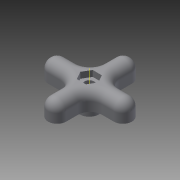
# Autodesk Inventor part: coil tightner
Saved by Autodesk Inventor 2013 (Build 170138000, 138)
## iProperties
Created: 2013-01-17
Part Number: coil tightner
Material: Generic
Document SubType Name: Modeling
Designer: Nico
Density: 1 g/cm^3
Author: Nico
Autodesk Inventor part; units mm, degrees
ref_plane "YZ Plane" through (0, 0, 0) normal (1, 0, 0) x (0, 1, 0)
ref_plane "XZ Plane" through (0, 0, 0) normal (0, 1, 0) x (-1, 0, 0)
ref_plane "XY Plane" through (0, 0, 0) normal (0, 0, 1) x (1, 0, 0)
sketch "Sketch1" plane through (0, 0, 0) normal (0, 0, 1) x (1, 0, 0)
  line L0 (17.5, 0) -> (27.5, 0)
  line L1 (35, 7.5) -> (35, 7.5)
  line L2 (27.5, 15) -> (17.5, 15)
  line L3 (0, 15) -> (0, 0)
  line L4 (-7.5, 7.5) -> (7.5, 7.5)
  line L5 (7.5, -10) -> (7.5, -20)
  line L6 (0, -27.5) -> (0, -27.5)
  line L7 (-7.5, -20) -> (-7.5, -10)
  line L8 (-17.5, 0) -> (-27.5, 0)
  line L9 (-35, 7.5) -> (-35, 7.5)
  line L10 (-27.5, 15) -> (-17.5, 15)
  line L11 (0, 15) -> (0, 0)
  line L12 (-7.5, 7.5) -> (7.5, 7.5)
  line L13 (7.5, 25) -> (7.5, 35)
  line L14 (0, 42.5) -> (0, 42.5)
  line L15 (-7.5, 35) -> (-7.5, 25)
  arc A0 (-17.5, 15) -> (-7.5, 25) centre (-17.5, 25) ccw
  arc A1 (7.5, 25) -> (17.5, 15) centre (17.5, 25) ccw
  arc A2 (17.5, 0) -> (7.5, -10) centre (17.5, -10) ccw
  arc A3 (-7.5, -10) -> (-17.5, 0) centre (-17.5, -10) ccw
  arc A4 (-27.5, 15) -> (-35, 7.5) centre (-27.5, 7.5) ccw
  arc A5 (-35, 7.5) -> (-27.5, 0) centre (-27.5, 7.5) ccw
  arc A6 (-7.5, -20) -> (0, -27.5) centre (0, -20) ccw
  arc A7 (0, -27.5) -> (7.5, -20) centre (0, -20) ccw
  arc A8 (27.5, 0) -> (35, 7.5) centre (27.5, 7.5) ccw
  arc A9 (35, 7.5) -> (27.5, 15) centre (27.5, 7.5) ccw
  arc A10 (7.5, 35) -> (0, 42.5) centre (0, 35) ccw
  arc A11 (0, 42.5) -> (-7.5, 35) centre (0, 35) ccw
  point P0 (35, 0)
  point P1 (7.5, -27.5)
  point P2 (-35, 0)
  point P3 (7.5, 42.5)
  dimension "d0" = 35
  dimension "d1" = 15
  dimension "d2" = 15
  dimension "d3" = 7.5
  dimension "d4" = 7.5
  dimension "d5" = 35
  dimension "d6" = 35
  dimension "d7" = 35
  dimension "d8" = 10
  dimension "d9" = 7.5
  constraints: 32 end point, 24 point on circle, 24 tangent, 16 point on line, 12 centre point, 10 equal radius, 8 parallel, 4 horizontal, 4 perpendicular
  measures "d0" distance of L3.end point (35, 0)
  measures "d1" distance of L3.start L3.end
  measures "d2" distance of L4.start L4.end
  measures "d3" distance between parallel lines of L5 L3
  measures "d4" distance between parallel lines of L0 L4
  measures "d5" distance of L4.end point (7.5, -27.5)
  measures "d6" distance of L3.end point (-35, 0)
  measures "d7" distance of L12.end point (7.5, 42.5)
  measures "d8" radius of A0
  measures "d9" radius of A4
extrude "Extrusion1" add sketch "Sketch1" along normal blind 15
sketch "Sketch2" plane through (0, 0, 15) normal (0, 0, 1) x (1, 0, 0)
  circle A0 centre (0, 6.9274) radius 3.95
  point P0 (0, 0)
  dimension "d12" = 7.9
  constraints: 1 centre point
  measures "d12" diameter of A0
extrude "Extrusion2" cut sketch "Sketch2" against normal blind 15
sketch "Sketch3" plane through (0, 0, 15) normal (0, 0, 1) x (1, 0, 0)
  circle A0 centre (0, 6.9274) radius 3.95 projected
  line L0 (-3.7206, 13.5785) -> (3.8997, 13.475)
  line L1 (3.8997, 13.475) -> (7.6203, 6.824)
  line L2 (7.6203, 6.824) -> (3.7206, 0.2763)
  line L3 (3.7206, 0.2763) -> (-3.8997, 0.3797)
  line L4 (-3.8997, 0.3797) -> (-7.6203, 7.0308)
  line L5 (-7.6203, 7.0308) -> (-3.7206, 13.5785)
  point P0 (0, 0)
  dimension "d16" = 13.2
  constraints: 12 end point, 1 coincident, 13 other
  measures "d16" distance between parallel lines of L3 L0
extrude "Extrusion3" cut sketch "Sketch3" against normal blind 5
sketch "Sketch4" plane through (0, 0, 0) normal (0, 0, -1) x (-1, 0, 0)
  circle A0 centre (0, 6.9274) radius 3.95 projected
  circle A1 centre (0, 6.9274) radius 8
  point P0 (0, 0)
  dimension "d19" = 16
  constraints: 1 centre point, 1 coincident
  measures "d19" diameter of A1
extrude "Extrusion4" add sketch "Sketch4" along normal blind 8
fillet "Fillet1" radius 3 1 edges at (8, 6.9274, 0)
fillet "Fillet2" radius 7.5 16 edges at (10.4289, 17.9289, 15) (7.5, 30, 15) (0, 42.5, 15) (-7.5, 30, 15) (-10.4289, 17.9289, 15) (-22.5, 15, 15) (-35, 7.5, 15) (-22.5, 0, 15) (-10.4289, -2.9289, 15) (-7.5, -15, 15) (0, -27.5, 15) (7.5, -15, 15) (10.4289, -2.9289, 15) (22.5, 0, 15) (35, 7.5, 15) (22.5, 15, 15)
body "Solid1"
